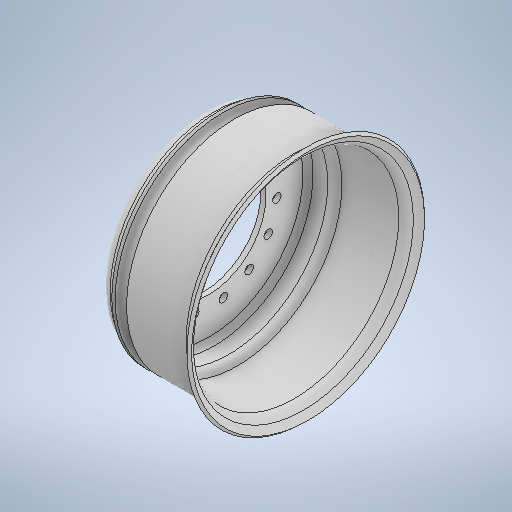
# Autodesk Inventor part: 24110246 wheel rim
Saved by Autodesk Inventor 2025 (Build 290162000, 162)
## iProperties
Created: 2024-11-05
Part Number: 24110246 wheel rim
Material: Generic
Document SubType Name: Modeling
Designer: DELL
Density: 1 g/cm^3
Appearance: Default
Author: DELL
Autodesk Inventor part; units mm, degrees
ref_plane "YZ Plane" through (0, 0, 0) normal (1, 0, 0) x (0, 1, 0)
ref_plane "XZ Plane" through (0, 0, 0) normal (0, 1, 0) x (-1, 0, 0)
ref_plane "XY Plane" through (0, 0, 0) normal (0, 0, 1) x (1, 0, 0)
sketch "Sketch1" plane through (0, 0, 0) normal (0, 0, 1) x (1, 0, 0)
  line L0 (0, 190) -> (6, 190)
  line L1 (26, 190) -> (131, 190)
  arc A0 (131, 190) -> (141.9127, 196.4038) centre (131, 202.5) ccw
  arc A1 (151, 208.9038) -> (141.9127, 196.4038) centre (198.6585, 164.7035) ccw
  arc A2 (6, 190) -> (26, 190) centre (16, 190) ccw
  arc A3 (155.3992, 204.8238) -> (147.1507, 193.4776) centre (198.6585, 164.7035) ccw
  arc A4 (131, 184) -> (147.1507, 193.4776) centre (131, 202.5) ccw
  line L2 (131, 184) -> (30.8324, 184)
  line L3 (1.1676, 184) -> (0, 184)
  line L4 (151, 208.9038) -> (155.3992, 204.8238)
  line L5 (16, 174) -> (-9.8999, 174)
  arc A5 (-9.8999, 174) -> (-18.8999, 165) centre (-9.8999, 165) ccw
  line L6 (-18.8999, 165) -> (-18.8999, 100)
  line L7 (-18.8999, 100) -> (-27.8999, 100)
  line L8 (-27.8999, 100) -> (-27.8999, 165)
  arc A6 (-9.8999, 183) -> (-27.8999, 165) centre (-9.8999, 165) ccw
  line L9 (1.6125, 183) -> (-9.8999, 183)
  line L10 (0, 190) -> (0, 184)
  arc A7 (1.1676, 184) -> (1.6125, 183) centre (16, 190) ccw
  arc A8 (16, 174) -> (30.8324, 184) centre (16, 190) ccw
  line L11 (0, 0) -> (39.9191, 0)
  point P0 (-4.1437, 183)
  point P1 (3, 190)
  dimension "d0" = 6
  dimension "d2" = 105
  dimension "d3" = 12.5
  dimension "d6" = 65
  dimension "d7" = 12.5
  dimension "d8" = 10
  dimension "d13" = 6
  dimension "d14" = 9
  dimension "d15" = 18
  dimension "d16" = 9
  dimension "d17" = 65
  dimension "d18" = 9
  dimension "d19" = 190
  constraints: 24 end point, 18 point on circle, 9 centre point, 7 tangent, 5 horizontal, 2 collinear, 2 midpoint, 2 vertical, 1 vertical alignment, 2 other
  measures "d0" distance of L0.start L0.end
  measures "d2" distance of L1.start L1.end
  measures "d3" radius of A0
  measures "d6" radius of A1
  measures "d7" vertical distance of L4.start A0.end
  measures "d8" radius of A2
  measures "d13" radial gap between concentric circles of A0 A4
  measures "d14" radius of A5
  measures "d15" radius of A6
  measures "d16" distance of L6.end L7.end
  measures "d17" distance of L7.end L8.end
  measures "d18" distance from line of L5 point (-4.144, 183)
  measures "d19" distance from line of L11 point (3, 190)
sketch "Sketch2" plane through (0, 0, 0) normal (0, 0, 1) x (1, 0, 0)
  point P0 (0, 0)
revolve "Revolution1" add sketch "Sketch1" angle 360 about axis through (0, 0, 0) along (1, 0, 0)
sketch "Sketch3" plane through (-27.8999, 0, 0) normal (-1, 0, 0) x (0, 0, 1)
  circle A0 centre (0, 120) radius 7.5
  point P0 (0, 0)
  dimension "d21" = 15
  dimension "d22" = 120
  constraints: 1 centre point
  measures "d21" diameter of A0
  measures "d22" distance of A0.centre point (0, 0)
extrude "Extrusion1" cut sketch "Sketch3" against normal through all
pattern_circular "Circular Pattern1" count 15 over 360 about axis through (-23.3999, 0, 0) along (1, 0, 0) of "Extrusion1"
body "Solid1"
